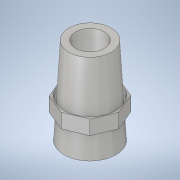
# Autodesk Inventor part: Tuerca_Conica
Saved by Autodesk Inventor 2020 (Build 240168000, 168)
## iProperties
Created: 2019-09-23
Part Number: Tuerca_Conica
Material: Genérico
Document SubType Name: Modeling
Designer: axelj
Density: 1 g/cm^3
Appearance: Aluminio - Pulido
Author: axelj
Autodesk Inventor part; units mm, degrees
ref_plane "YZ Plane" through (0, 0, 0) normal (1, 0, 0) x (0, 1, 0)
sketch "Boceto1" plane through (0, 0, 0) normal (0, 1, 0) x (-1, 0, 0)
  circle A0 centre (0, 0) radius 2.7
  circle A1 centre (0, 0) radius 1.5
  dimension "d0" = 5.4
  dimension "d1" = 3
  constraints: 2 centre point, 2 coincident
  measures "d0" diameter of A0
  measures "d1" diameter of A1
ref_plane "Plano de trabajo1" through (0, 9, 0) normal (0, 1, 0) x (-1, 0, 0)
sketch "Boceto2" plane through (0, 9, 0) normal (0, 1, 0) x (-1, 0, 0)
  circle A0 centre (0, 0) radius 1.5
  circle A1 centre (0, 0) radius 2.2
  dimension "d3" = 3
  dimension "d4" = 4.4
  constraints: 2 centre point, 2 coincident
  measures "d3" diameter of A0
  measures "d4" diameter of A1
sketch "Boceto3" plane through (0, 0, 0) normal (0, 0, 1) x (1, 0, 0)
  point P0 (0, 0)
loft "Solevación1" add profiles "Boceto1", "Boceto2" contours A0 | A1 / A0 | A1
sketch "Boceto4" plane through (0, 0, 0) normal (0, 1, 0) x (-1, 0, 0)
  circle A0 centre (0, 0) radius 1.5
  dimension "d10" = 3
  constraints: 1 centre point, 1 coincident
  measures "d10" diameter of A0
extrude "Extrusión1" cut sketch "Boceto4" along normal blind 10
ref_plane "Plano de trabajo2" through (0, 4, 0) normal (0, 1, 0) x (-1, 0, 0)
sketch "Boceto5" plane through (0, 4, 0) normal (0, 1, 0) x (-1, 0, 0)
  line L0 (-3, 0.0004) -> (1, 0.0004) construction
  circle A0 centre (0, 0) radius 2.7 projected
  line L1 (0, 2.7) -> (-2.7, 0)
  line L2 (0, -2.7) -> (-2.7, 0)
  line L3 (0, -2.7) -> (2.7, 0)
  line L4 (2.7, 0) -> (0, 2.7)
  line L5 (3.2285, -3.2285) -> (7.2285, -3.2285) construction
  line L6 (2.1213, -2.1213) -> (3, 0.0004)
  line L7 (3, 0.0004) -> (2.0975, 2.1448)
  line L8 (-2.0969, -2.1454) -> (-3, 0.0004)
  line L9 (-3, 0.0004) -> (-2.1213, 2.1213)
  line L10 (-0.0004, -3) -> (2.1213, -2.1213)
  line L11 (-2.0969, -2.1454) -> (-0.0004, -3)
  line L12 (-2.1213, 2.1213) -> (-0.0004, 3)
  line L13 (-0.0004, 3) -> (2.0975, 2.1448)
  circle A1 centre (0, 0) radius 1.5
  dimension "d33" = 3
  constraints: 28 end point, 4 point on circle, 3 perpendicular, 2 horizontal, 2 parallel, 1 centre point, 1 coincident
  measures "d33" diameter of A1
extrude "Extrusión2" add sketch "Boceto5" against normal blind 1.5 contours L10 L11 L8 L9 L12 L13 L7 L6
